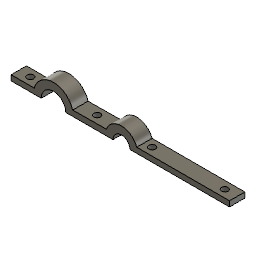
Trumpet+Mount+Close+Top (Autodesk Fusion 360 design; units mm, degrees)
Autodesk Fusion 360 part; units mm, degrees
sketch "Sketch1" plane through (0, 0, 0) normal (0, 0, 1) x (1, 0, 0)
  circle A0 centre (-43.925, 0) radius 12.925
  circle A1 centre (-43.925, 0) radius 7.925
  circle A2 centre (0, 0) radius 10.5
  circle A3 centre (0, 0) radius 5.5
  line L0 (9.8995, 3.5) -> (69.8995, 3.5)
  line L1 (69.8995, 3.5) -> (69.8995, -3.5)
  line L2 (69.8995, -3.5) -> (9.8995, -3.5)
  line L3 (-31.5162, 3.6163) -> (-9.7806, 3.8197)
  line L4 (-31.4507, -3.3834) -> (-10.006, -3.1827)
  line L5 (-56.3671, 3.5) -> (-71.3671, 3.5)
  line L6 (-71.3671, 3.5) -> (-71.3671, -3.5)
  line L7 (-71.3671, -3.5) -> (-56.3671, -3.5)
  line L8 (-43.925, 0) -> (0, 0) construction
  dimension "d1" = 3.5
  dimension "d2" = 3.5
  dimension "d3" = 3.5
  dimension "d4" = 3.5
  dimension "d5" = 3.5
  dimension "d6" = 3.5
  dimension "d7" = 43.925
  dimension "d8" = 60
  dimension "d9" = 15
  dimension "d19" = 25.85
  dimension "d20" = 21
  dimension "d21" = 11
  dimension "d22" = 15.85
  constraint concentric A0 A1
  constraint concentric A2 A3
  constraint coincident A2 L0.start
  constraint horizontal L0
  constraint perpendicular L0 L1
  constraint coincident A2 L2.end
  constraint perpendicular L1 L2
  constraint coincident A0 L3.start
  constraint coincident A2 L3.end
  constraint coincident A0 L4.start
  constraint coincident A2 L4.end
  constraint parallel L3 L4
  constraint coincident A0 L5.start
  constraint horizontal L5
  constraint perpendicular L5 L6
  constraint coincident A0 L7.end
  constraint perpendicular L6 L7
  constraint coincident A0.centre A1.centre
  constraint coincident A2.centre A3.centre
  constraint horizontal L8
  measures "d1" distance of A2.centre L2
  measures "d2" distance of A2.centre L0
  measures "d3" distance of A0.centre L3
  measures "d4" distance of A0.centre L4
  measures "d5" distance of A0.centre L7
  measures "d6" distance of A0.centre L5
  measures "d7" horizontal distance of A0.centre A2.centre
  measures "d8" distance of L0.start L0.end
  measures "d9" distance of L5.start L5.end
  measures "d19" diameter of A0
  measures "d20" diameter of A2
  measures "d21" diameter of A3
  measures "d22" diameter of A1
extrude "Extrude1" add sketch "Sketch1" along normal mid plane 10
sketch "Sketch4" plane through (0, 3.5, 0) normal (0, 1, 0) x (-1, 0, 0)
  line L0 (71.3671, -5) -> (71.3671, 5)
  line L1 (71.3671, 5) -> (56.3671, 5)
  line L2 (56.3671, 5) -> (56.3671, -5)
  line L3 (56.3671, -5) -> (71.3671, -5)
  circle A0 centre (63.8671, 0) radius 2.125
  line L4 (31.5162, -5) -> (9.7806, -5)
  line L5 (31.5162, 5) -> (31.5162, -5)
  line L6 (9.7806, -5) -> (9.7806, 5)
  dimension "d25" = 4.25
  dimension "d27" = 5
  dimension "d31" = 7.5
  dimension "d32" = 7.5
  measures "d25" diameter of A0
  measures "d27" distance of L3 A0.centre
  measures "d31" distance of L0 A0.centre
  measures "d32" distance of L2 A0.centre
extrude "Extrude4" cut sketch "Sketch4" along normal up to surface contours A0 end surface through (-31.4507, -3.3834, 0) normal (0.009359, -0.999956, 0) offset 0
sketch "Sketch5" plane through (-0.0366, 3.9109, 0) normal (-0.009359, 0.999956, 0) x (0, 0, 1)
  line L0 (-5, -31.481) -> (5, -31.481)
  line L1 (5, -31.481) -> (5, -9.7444)
  line L2 (5, -9.7444) -> (-5, -9.7444)
  line L3 (-5, -9.7444) -> (-5, -31.481)
  circle A0 centre (0, -20.613) radius 2.125
  dimension "d35" = 4.25
  dimension "d36" = 10.868
  dimension "d37" = 10.8686
  dimension "d38" = 5
  measures "d35" diameter of A0
  measures "d36" distance of L0 A0.centre
  measures "d37" distance of L2 A0.centre
  measures "d38" distance of L3 A0.centre
extrude "Extrude5" cut sketch "Sketch5" against normal up to surface (7 mm away) contours A0
sketch "Sketch6" plane through (0, 3.5, 0) normal (0, 1, 0) x (-1, 0, 0)
  line L0 (-9.8995, -5) -> (-9.8995, 5)
  line L1 (-9.8995, 5) -> (-69.8995, 5)
  line L2 (-69.8995, 5) -> (-69.8995, -5)
  line L3 (-69.8995, -5) -> (-9.8995, -5)
sketch "Sketch7" plane through (0, 3.5, 0) normal (0, 1, 0) x (-1, 0, 0)
  line L0 (-9.8995, -5) -> (-9.8995, 5) construction
  line L1 (-9.8995, 5) -> (-69.8995, 5) construction
  line L2 (-69.8995, 5) -> (-69.8995, -5) construction
  line L3 (-69.8995, -5) -> (-9.8995, -5) construction
  line L4 (-69.8995, 0) -> (-9.8995, 0) construction
  circle A0 centre (-61.8995, 0) radius 2.125
  circle A1 centre (-14.8995, 0) radius 2.125
  dimension "d41" = 4.25
  dimension "d42" = 4.25
  dimension "d43" = 8
  dimension "d44" = 5
  constraint midpoint L2 L4.start
  constraint midpoint L0 L4.end
  constraint coincident L4 A0.centre
  constraint coincident L4 A1.centre
  measures "d41" diameter of A0
  measures "d42" diameter of A1
  measures "d43" distance of L2 A0.centre
  measures "d44" distance of L0 A1.centre
extrude "Extrude6" cut sketch "Sketch7" against normal up to surface (7 mm away)
sketch "Sketch3" plane through (0, 0, 0) normal (0, 1, 0) x (1, 0, 0)
  line L0 (-71.3671, 5) -> (-71.3671, -5)
  line L1 (-71.3671, -5) -> (-56.3671, -5)
  line L2 (-56.3671, -5) -> (-56.3671, 5)
  line L3 (-56.3671, 5) -> (-71.3671, 5)
  line L4 (9.8995, 5) -> (9.8995, -5)
  line L5 (9.8995, -5) -> (69.8995, -5)
  line L6 (69.8995, -5) -> (69.8995, 5)
  line L7 (69.8995, 5) -> (9.8995, 5)
  line L8 (-71.3671, 5) -> (69.8995, 5)
  line L9 (69.8995, 5) -> (69.8995, -5)
  line L10 (69.8995, -5) -> (-71.3671, -5)
  line L11 (-71.3671, -5) -> (-71.3671, 5)
  circle A0 centre (-63.8671, 0) radius 2.125
  circle A1 centre (14.8995, 0) radius 2.125
  circle A2 centre (61.8995, 0) radius 2.125
  constraint horizontal L8
  constraint vertical L9
  constraint horizontal L10
  constraint vertical L11
  constraint coincident L5.end L6.start
  constraint coincident L0.start L3.end
extrude "Extrude3" cut sketch "Sketch3" against normal blind 20 contours L0 L1 L2 L3 L8 L10 L11 | L2 L4 L8 L10 | L4 L5 L6 L7 L8 L9 L10 | A0 | A1 | A2
equation "d2 = d1"
equation "d3 = d1"
equation "d4 = d1"
equation "d5 = d1"
equation "d6 = d1"
equation "d42 = d41"
